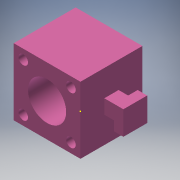
# Autodesk Inventor part: capuchon_roulement
Saved by Autodesk Inventor 2017 (Build 210142000, 142)
## iProperties
Created: 2017-12-27
Part Number: capuchon_roulement
Material: Generic
Document SubType Name: Modeling
Designer: franc
Density: 1 g/cm^3
Appearance: Default
Author: franc
Autodesk Inventor part; units mm, degrees
ref_plane "YZ Plane" through (0, 0, 0) normal (1, 0, 0) x (0, 1, 0)
ref_plane "XZ Plane" through (0, 0, 0) normal (0, 1, 0) x (-1, 0, 0)
ref_plane "XY Plane" through (0, 0, 0) normal (0, 0, 1) x (1, 0, 0)
sketch "Esquisse1" plane through (0, 0, 0) normal (0, 1, 0) x (-1, 0, 0)
  line L0 (4.4286, 5.3714) -> (-9.5714, 5.3714)
  line L1 (-9.5714, 5.3714) -> (-9.5714, -8.6286)
  line L2 (-9.5714, -8.6286) -> (4.4286, -8.6286)
  line L3 (4.4286, -8.6286) -> (4.4286, 5.3714)
  point P0 (0, 0)
  dimension "d0" = 14
  dimension "d1" = 14
  constraints: 8 end point, 2 parallel, 1 horizontal, 1 perpendicular
  measures "d0" distance of L2.end L0.start
  measures "d1" distance of L0.start L0.end
extrude "Extrusion1" add sketch "Esquisse1" along normal blind 13
sketch "Esquisse2" plane through (0, 0, 0) normal (0, -1, 0) x (1, 0, 0)
  circle A0 centre (2.5714, -1.6286) radius 4
  line L0 (-4.4286, 5.3714) -> (9.5714, 5.3714) projected
  line L1 (9.5714, 5.3714) -> (9.5714, -8.6286) projected
  point P0 (0, 0)
  dimension "d4" = 7
  dimension "d5" = 7
  dimension "d6" = 8
  constraints: 1 centre point
  measures "d4" distance from line of L0 A0.centre
  measures "d5" distance from line of L1 A0.centre
  measures "d6" diameter of A0
extrude "Extrusion2" cut sketch "Esquisse2" against normal blind 12
sketch "Esquisse3" plane through (2.5714, 12, -1.6286) normal (0, -1, 0) x (1, 0, 0)
  circle A0 centre (0, 0) radius 2.5
  line L0 (7, -7) -> (-7, -7) projected
  line L1 (7, 7) -> (7, -7) projected
  point P0 (-2.5714, 1.6286)
  dimension "d9" = 5
  dimension "d10" = 7
  dimension "d11" = 7
  constraints: 1 centre point
  measures "d9" diameter of A0
  measures "d10" distance from line of L0 A0.centre
  measures "d11" distance from line of L1 A0.centre
extrude "Extrusion3" cut sketch "Esquisse3" against normal through all
sketch "Esquisse4" plane through (0, 0, 0) normal (0, -1, 0) x (1, 0, 0)
  circle A0 centre (7.5714, 3.3714) radius 1
  circle A1 centre (-2.4286, 3.3714) radius 1
  circle A2 centre (-2.4286, -6.6286) radius 1
  circle A3 centre (7.5714, -6.6286) radius 1
  line L0 (-4.4286, -8.6286) -> (-4.4286, 5.3714) projected
  line L1 (-4.4286, 5.3714) -> (9.5714, 5.3714) projected
  line L2 (9.5714, 5.3714) -> (9.5714, -8.6286) projected
  line L3 (9.5714, -8.6286) -> (-4.4286, -8.6286) projected
  point P0 (0, 0)
  dimension "d14" = 2
  dimension "d15" = 2
  dimension "d16" = 2
  dimension "d17" = 2
  dimension "d19" = 2
  dimension "d20" = 2
  dimension "d21" = 2
  dimension "d22" = 2
  dimension "d23" = 2
  dimension "d24" = 2
  dimension "d25" = 2
  dimension "d26" = 2
  constraints: 4 centre point
  measures "d14" diameter of A0
  measures "d15" diameter of A3
  measures "d16" diameter of A2
  measures "d17" diameter of A1
  measures "d19" distance from line of L1 A0.centre
  measures "d20" distance from line of L2 A0.centre
  measures "d21" distance from line of L2 A3.centre
  measures "d22" distance from line of L3 A3.centre
  measures "d23" distance from line of L3 A2.centre
  measures "d24" distance from line of L0 A2.centre
  measures "d25" distance from line of L0 A1.centre
  measures "d26" distance from line of L1 A1.centre
extrude "Extrusion4" cut sketch "Esquisse4" against normal through all contours A0 | A1 | A2 | A3
sketch "Esquisse5" plane through (9.5714, 0, 5.3714) normal (1, 0, 0) x (0, 0, -1)
  point P0 (5.3714, 0)
sketch "Esquisse6" plane through (9.5714, 0, 5.3714) normal (1, 0, 0) x (0, 0, -1)
  line L0 (5.5, 8) -> (8.5, 8)
  line L1 (8.5, 8) -> (8.5, 5)
  line L2 (8.5, 5) -> (5.5, 5)
  line L3 (5.5, 5) -> (5.5, 8)
  line L4 (0, 0) -> (0, 13) projected
  line L5 (0, 13) -> (14, 13) projected
  point P0 (5.3714, 0)
  dimension "d29" = 3
  dimension "d30" = 3
  dimension "d31" = 5.5
  dimension "d32" = 5
  constraints: 8 end point, 2 parallel, 1 horizontal, 1 perpendicular
  measures "d29" distance of L0.start L0.end
  measures "d30" distance of L2.end L0.start
  measures "d31" distance between parallel lines of L4 L3
  measures "d32" distance between parallel lines of L5 L0
extrude "Extrusion5" add sketch "Esquisse6" along normal blind 3
sketch "Esquisse7" plane through (12.5714, 0, 5.3714) normal (1, 0, 0) x (0, 0, -1)
  line L0 (4.5, 9) -> (9.5, 9)
  line L1 (9.5, 9) -> (9.5, 4)
  line L2 (9.5, 4) -> (4.5, 4)
  line L3 (4.5, 4) -> (4.5, 9)
  line L4 (0, 13) -> (14, 13) projected
  line L5 (0, 0) -> (0, 13) projected
  point P0 (5.3714, 0)
  dimension "d35" = 5
  dimension "d36" = 5
  dimension "d37" = 4
  dimension "d38" = 4.5
  constraints: 8 end point, 2 parallel, 1 horizontal, 1 perpendicular
  measures "d35" distance of L2.end L0.start
  measures "d36" distance of L0.start L0.end
  measures "d37" distance between parallel lines of L4 L0
  measures "d38" distance between parallel lines of L5 L3
extrude "Extrusion6" add sketch "Esquisse7" along normal blind 2
